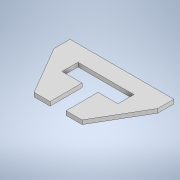
# Autodesk Inventor part: Latch Clip
Saved by Autodesk Inventor 2022.2 (Build 262287030, 287C)
## iProperties
Created: 2023-02-22
Part Number: Latch Clip
Material: Generic
Document SubType Name: Modeling
Designer: jak27277
Density: 1 g/cm^3
Appearance: Default
Author: jak27277
Autodesk Inventor part; units mm, degrees
ref_plane "YZ Plane" through (0, 0, 0) normal (1, 0, 0) x (0, 1, 0)
ref_plane "XZ Plane" through (0, 0, 0) normal (0, 1, 0) x (-1, 0, 0)
ref_plane "XY Plane" through (0, 0, 0) normal (0, 0, 1) x (1, 0, 0)
sketch "Sketch1" plane through (0, 0, 0) normal (0, 1, 0) x (-1, 0, 0)
  line L0 (82.55, 0) -> (-82.55, 0)
  line L1 (-82.55, 0) -> (-82.55, 0.0715)
  line L2 (-82.55, 0.0715) -> (-82.55, 25.4)
  line L3 (-38.1, 101.6) -> (-12.7, 101.6)
  line L4 (-12.7, 101.6) -> (-12.7, 50.8)
  line L5 (-12.7, 50.8) -> (-44.45, 50.8)
  line L6 (-44.45, 50.8) -> (-44.45, 25.4)
  line L7 (-44.45, 25.4) -> (44.45, 25.4)
  line L8 (44.45, 25.4) -> (44.45, 50.8)
  line L9 (38.1, 101.6) -> (82.55, 25.4)
  line L10 (82.55, 25.4) -> (82.55, 0)
  line L11 (38.1, 101.6) -> (12.7, 101.6)
  line L12 (12.7, 101.6) -> (12.7, 50.8)
  line L13 (12.7, 50.8) -> (44.45, 50.8)
  line L14 (0, 0) -> (0, 111.0493) construction
  line L15 (-82.55, 25.4) -> (-38.1, 101.6)
  point P0 (82.55, 12.7)
  dimension "d0" = 165.1
  dimension "d3" = 38.1
  dimension "d4" = 25.4
  dimension "d5" = 25.4
  dimension "d6" = 101.6
  dimension "d7" = 44.45
  dimension "d8" = 69.85
  dimension "d9" = 120.65
  dimension "d10" = 25.4
  dimension "d11" = 88.9
  dimension "d12" = 25.4
  constraints: 32 end point, 9 perpendicular, 3 point on line, 2 coincident, 2 horizontal, 2 midpoint, 2 vertical, 1 parallel, 1 other
  measures "d0" distance of L0.start L0.end
  measures "d3" distance from line of point (82.55, 12.7) L8
  measures "d4" distance between parallel lines of L0 L7
  measures "d5" distance of L5.end L6.end
  measures "d6" distance between parallel lines of L11 L0
  measures "d7" horizontal distance of L9.start L9.end
  measures "d8" distance between parallel lines of L12 L10
  measures "d9" distance from line of L3.start L10
  measures "d10" distance between parallel lines of L12 L4
  measures "d11" distance of L6.end L7.end
  measures "d12" distance of L9.end L0.start
extrude "Extrusion1" add sketch "Sketch1" along normal blind 6.35
body "Solid1"
